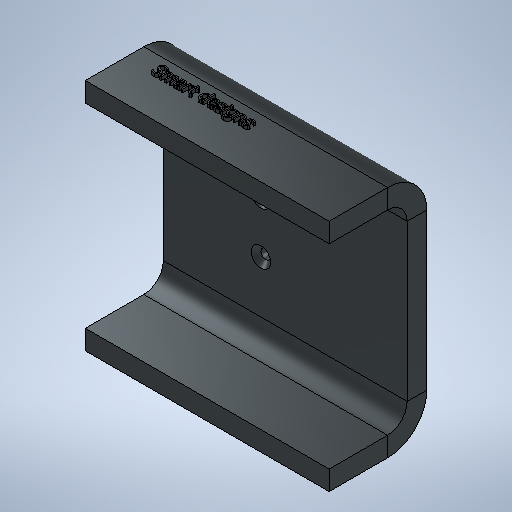
# Autodesk Inventor part: base
Saved by Autodesk Inventor 2025 (Build 290162010, 162A)
## iProperties
Created: 2024-06-06
Part Number: base
Material: Iron, Gray
Document SubType Name: Sheet Metal
Designer: ffogue
Density: 7.15 g/cm^3
Sheet Metal Rule: Default_mm
Appearance: Iron Gray
Author: ffogue
Autodesk Inventor part; units mm, degrees
note: some values were not read from the file. Chosen so that the rebuilt part matches the saved one: direction of "Bohrung2"; direction of "Emboss1".
ref_plane "YZ Plane" through (0, 0, 0) normal (1, 0, 0) x (0, 1, 0)
ref_plane "XZ Plane" through (0, 0, 0) normal (0, 1, 0) x (-1, 0, 0)
ref_plane "XY Plane" through (0, 0, 0) normal (0, 0, 1) x (1, 0, 0)
sketch "Skizze1" plane through (0, 0, 0) normal (0, 1, 0) x (-1, 0, 0)
  line L0 (37.5, -30) -> (-37.5, -30)
  line L1 (-37.5, -30) -> (-37.5, 30)
  line L2 (-37.5, 30) -> (37.5, 30)
  line L3 (37.5, 30) -> (37.5, -30)
  line L4 (37.5, -30) -> (-37.5, 30) construction
  line L5 (-37.5, -30) -> (37.5, 30) construction
  point P0 (0, 0)
  dimension "d0" = 75
  dimension "d1" = 60
  measures "d0" distance between parallel lines of L3 L1
  measures "d1" distance between parallel lines of L0 L2
extrude "Grobblech2" add sketch "Skizze1" along normal blind 6
sketch "Skizze2" plane through (-37.5, 0, -30) normal (0, 0, -1) x (-1, 0, 0)
  line L0 (-75, 0) -> (0, 0)
  line L1 (0, 0) -> (0, 24)
  line L2 (0, 24) -> (-75, 24)
  line L3 (-75, 24) -> (-75, 0)
  constraints: 6 end point, 1 horizontal, 1 perpendicular, 1 vertical
edge flange "Lasche1" height 30 angle 90 thickness 6 bend radius 6 thickness toward (0, 0, -1) relief tear relief width 6 relief depth 3 corner gap 6 corner form 0 edges at (0, 6, -30) (0, 6, 30) wall of the first edge with corners at (37.5, 0, -30) (-37.5, 0, -30) (-37.5, -24, -30) (37.5, -24, -30)
bend "Biegung1"
corner "Ecke1"
sketch "Skizze3" plane through (0, 0, 0) normal (0, 1, 0) x (1, 0, 0)
  line L0 (-37.5, -24) -> (-37.5, 24) projected
  line L1 (-37.5, 36) -> (37.5, 36) projected
  line L2 (-37.5, 24) -> (-37.5, 36) projected
  line L3 (37.5, 24) -> (-37.5, 24) projected
  line L4 (37.5, 24) -> (37.5, 36) projected
  point P0 (0, 0)
  point P1 (-7.5, 8)
  point P2 (-7.5, -8)
  dimension "d23" = 16
  dimension "d24" = 30
  dimension "d25" = 28
  constraints: 1 vertical alignment
  measures "d23" distance of point (-7.5, -8) point (-7.5, 8)
  measures "d24" distance from line of L0 point (-7.5, 8)
  measures "d25" distance from line of point (-7.5, 8) L1
hole "Bohrung2" at (-7.5, 0, -8) at (-7.5, 0, 8) direction (0, 1, 0) diameter 3 end up to surface countersink diameter 6 countersink angle 90
sketch "Sketch4" plane through (-37.5, -24, 36) normal (0, 0, 1) x (1, 0, 0)
  line L0 (8.2536, 15.3295) -> (38.2844, 15.3295) construction
  line L1 (38.2844, 15.3295) -> (38.2844, 10.6808) construction
  line L2 (38.2844, 10.6808) -> (8.2536, 10.6808) construction
  line L3 (8.2536, 10.6808) -> (8.2536, 15.3295) construction
  spline S0 degree 2 poles (9.5839, 11.6111) (9.2038, 11.6111) (8.6706, 11.77) (8.4352, 11.8834) knots 0 0 0 1 2 2 2
  line L4 (8.4352, 11.8834) -> (8.4352, 12.4677)
  line L5 (8.4352, 12.4677) -> (8.4692, 12.4677)
  spline S1 degree 2 poles (8.4692, 12.4677) (8.6989, 12.2521) (9.2804, 12.0139) (9.5498, 12.0139) knots 0 0 0 1 2 2 2
  spline S2 degree 2 poles (9.5498, 12.0139) (9.9356, 12.0139) (10.3298, 12.3344) (10.3298, 12.5982) knots 0 0 0 1 2 2 2
  spline S3 degree 2 poles (10.3298, 12.5982) (10.3298, 12.8081) (10.1228, 13.069) (9.8987, 13.1342) knots 0 0 0 1 2 2 2
  spline S4 degree 2 poles (9.8987, 13.1342) (9.737, 13.1796) (9.4676, 13.242) (9.2662, 13.2931) knots 0 0 0 1 2 2 2
  spline S5 degree 2 poles (9.2662, 13.2931) (9.0847, 13.3413) (8.7982, 13.4859) (8.6876, 13.6022) knots 0 0 0 1 2 2 2
  spline S6 degree 2 poles (8.6876, 13.6022) (8.5798, 13.7185) (8.4607, 14.0305) (8.4607, 14.2347) knots 0 0 0 1 2 2 2
  spline S7 degree 2 poles (8.4607, 14.2347) (8.4607, 14.6602) (9.1244, 15.2359) (9.6378, 15.2359) knots 0 0 0 1 2 2 2
  spline S8 degree 2 poles (9.6378, 15.2359) (9.9327, 15.2359) (10.4546, 15.1196) (10.6787, 15.009) knots 0 0 0 1 2 2 2
  line L6 (10.6787, 15.009) -> (10.6787, 14.4531)
  line L7 (10.6787, 14.4531) -> (10.6446, 14.4531)
  spline S9 degree 2 poles (10.6446, 14.4531) (10.4773, 14.6063) (9.9554, 14.8332) (9.669, 14.8332) knots 0 0 0 1 2 2 2
  spline S10 degree 2 poles (9.669, 14.8332) (9.3456, 14.8332) (8.9457, 14.5297) (8.9457, 14.2829) knots 0 0 0 1 2 2 2
  spline S11 degree 2 poles (8.9457, 14.2829) (8.9457, 14.0617) (9.1811, 13.7979) (9.4023, 13.7384) knots 0 0 0 1 2 2 2
  spline S12 degree 2 poles (9.4023, 13.7384) (9.5498, 13.6987) (9.9781, 13.5966) (10.1199, 13.554) knots 0 0 0 1 2 2 2
  spline S13 degree 2 poles (10.1199, 13.554) (10.4801, 13.4434) (10.8148, 12.9981) (10.8148, 12.6719) knots 0 0 0 1 2 2 2
  spline S14 degree 2 poles (10.8148, 12.6719) (10.8148, 12.4649) (10.6475, 12.0678) (10.4972, 11.9288) knots 0 0 0 1 2 2 2
  spline S15 degree 2 poles (10.4972, 11.9288) (10.3298, 11.7756) (9.9044, 11.6111) (9.5839, 11.6111) knots 0 0 0 1 2 2 2
  line L8 (14.2326, 11.6735) -> (14.2326, 13.1938)
  spline S16 degree 2 poles (14.2326, 13.1938) (14.2326, 13.3753) (14.2042, 13.6845) (14.1588, 13.7696) knots 0 0 0 1 2 2 2
  spline S17 degree 2 poles (14.1588, 13.7696) (14.1134, 13.8632) (13.9404, 13.9539) (13.7901, 13.9539) knots 0 0 0 1 2 2 2
  spline S18 degree 2 poles (13.7901, 13.9539) (13.654, 13.9539) (13.342, 13.7866) (13.1775, 13.6278) knots 0 0 0 1 2 2 2
  spline S19 degree 2 poles (13.1775, 13.6278) (13.1803, 13.588) (13.186, 13.4774) (13.186, 13.4037) knots 0 0 0 1 2 2 2
  line L9 (13.186, 13.4037) -> (13.186, 11.6735)
  line L10 (13.186, 11.6735) -> (12.7435, 11.6735)
  line L11 (12.7435, 11.6735) -> (12.7435, 13.1938)
  spline S20 degree 2 poles (12.7435, 13.1938) (12.7435, 13.3753) (12.7151, 13.6845) (12.6698, 13.7696) knots 0 0 0 1 2 2 2
  spline S21 degree 2 poles (12.6698, 13.7696) (12.6244, 13.8632) (12.4514, 13.9539) (12.301, 13.9539) knots 0 0 0 1 2 2 2
  spline S22 degree 2 poles (12.301, 13.9539) (12.1592, 13.9539) (11.8444, 13.7752) (11.6969, 13.6363) knots 0 0 0 1 2 2 2
  line L12 (11.6969, 13.6363) -> (11.6969, 11.6735)
  line L13 (11.6969, 11.6735) -> (11.2544, 11.6735)
  line L14 (11.2544, 11.6735) -> (11.2544, 14.3)
  line L15 (11.2544, 14.3) -> (11.6969, 14.3)
  line L16 (11.6969, 14.3) -> (11.6969, 14.0107)
  spline S23 degree 2 poles (11.6969, 14.0107) (11.8699, 14.1837) (12.2103, 14.3737) (12.4145, 14.3737) knots 0 0 0 1 2 2 2
  spline S24 degree 2 poles (12.4145, 14.3737) (12.6471, 14.3737) (13.0073, 14.161) (13.1009, 13.9199) knots 0 0 0 1 2 2 2
  spline S25 degree 2 poles (13.1009, 13.9199) (13.3023, 14.144) (13.6823, 14.3737) (13.9036, 14.3737) knots 0 0 0 1 2 2 2
  spline S26 degree 2 poles (13.9036, 14.3737) (14.0737, 14.3737) (14.3517, 14.2688) (14.4538, 14.1496) knots 0 0 0 1 2 2 2
  spline S27 degree 2 poles (14.4538, 14.1496) (14.5587, 14.0305) (14.675, 13.6731) (14.675, 13.4037) knots 0 0 0 1 2 2 2
  line L17 (14.675, 13.4037) -> (14.675, 11.6735)
  line L18 (14.675, 11.6735) -> (14.2326, 11.6735)
  spline S28 degree 2 poles (16.7597, 11.9515) (16.7058, 11.9118) (16.5243, 11.77) (16.4392, 11.7274) knots 0 0 0 1 2 2 2
  spline S29 degree 2 poles (16.4392, 11.7274) (16.3229, 11.665) (16.1045, 11.5998) (15.906, 11.5998) knots 0 0 0 1 2 2 2
  spline S30 degree 2 poles (15.906, 11.5998) (15.7443, 11.5998) (15.4522, 11.7218) (15.3416, 11.8324) knots 0 0 0 1 2 2 2
  spline S31 degree 2 poles (15.3416, 11.8324) (15.2366, 11.9402) (15.109, 12.2578) (15.109, 12.4337) knots 0 0 0 1 2 2 2
  spline S32 degree 2 poles (15.109, 12.4337) (15.109, 12.706) (15.3387, 13.0917) (15.5883, 13.2023) knots 0 0 0 1 2 2 2
  spline S33 degree 2 poles (15.5883, 13.2023) (15.8096, 13.3044) (16.4108, 13.381) (16.7597, 13.4008) knots 0 0 0 1 2 2 2
  line L19 (16.7597, 13.4008) -> (16.7597, 13.4859)
  spline S34 degree 2 poles (16.7597, 13.4859) (16.7597, 13.6391) (16.6661, 13.8291) (16.581, 13.883) knots 0 0 0 1 2 2 2
  spline S35 degree 2 poles (16.581, 13.883) (16.4959, 13.9369) (16.252, 13.9709) (16.1215, 13.9709) knots 0 0 0 1 2 2 2
  spline S36 degree 2 poles (16.1215, 13.9709) (15.9684, 13.9709) (15.5543, 13.8802) (15.3472, 13.7923) knots 0 0 0 1 2 2 2
  line L20 (15.3472, 13.7923) -> (15.3217, 13.7923)
  line L21 (15.3217, 13.7923) -> (15.3217, 14.2432)
  spline S37 degree 2 poles (15.3217, 14.2432) (15.4437, 14.2773) (15.9003, 14.3624) (16.1244, 14.3624) knots 0 0 0 1 2 2 2
  spline S38 degree 2 poles (16.1244, 14.3624) (16.3967, 14.3624) (16.7682, 14.2773) (16.9157, 14.1667) knots 0 0 0 1 2 2 2
  spline S39 degree 2 poles (16.9157, 14.1667) (17.0604, 14.0589) (17.2022, 13.7157) (17.2022, 13.4689) knots 0 0 0 1 2 2 2
  line L22 (17.2022, 13.4689) -> (17.2022, 11.6735)
  line L23 (17.2022, 11.6735) -> (16.7597, 11.6735)
  line L24 (16.7597, 11.6735) -> (16.7597, 11.9515)
  line L25 (16.7597, 12.3202) -> (16.7597, 13.0491)
  spline S40 degree 2 poles (16.7597, 13.0491) (16.6009, 13.035) (16.1215, 12.9867) (15.9712, 12.9414) knots 0 0 0 1 2 2 2
  spline S41 degree 2 poles (15.9712, 12.9414) (15.7954, 12.8875) (15.5656, 12.6634) (15.5656, 12.4649) knots 0 0 0 1 2 2 2
  spline S42 degree 2 poles (15.5656, 12.4649) (15.5656, 12.238) (15.8209, 12.0082) (16.0648, 12.0082) knots 0 0 0 1 2 2 2
  spline S43 degree 2 poles (16.0648, 12.0082) (16.2719, 12.0082) (16.6122, 12.1869) (16.7597, 12.3202) knots 0 0 0 1 2 2 2
  line L26 (19.216, 13.8263) -> (19.1933, 13.8263)
  spline S44 degree 2 poles (19.1933, 13.8263) (19.1422, 13.8405) (19.0316, 13.8461) (18.955, 13.8461) knots 0 0 0 1 2 2 2
  spline S45 degree 2 poles (18.955, 13.8461) (18.7763, 13.8461) (18.4246, 13.6902) (18.2658, 13.537) knots 0 0 0 1 2 2 2
  line L27 (18.2658, 13.537) -> (18.2658, 11.6735)
  line L28 (18.2658, 11.6735) -> (17.8233, 11.6735)
  line L29 (17.8233, 11.6735) -> (17.8233, 14.3)
  line L30 (17.8233, 14.3) -> (18.2658, 14.3)
  line L31 (18.2658, 14.3) -> (18.2658, 13.9085)
  spline S46 degree 2 poles (18.2658, 13.9085) (18.5069, 14.1241) (18.8671, 14.3) (19.0373, 14.3) knots 0 0 0 1 2 2 2
  spline S47 degree 2 poles (19.0373, 14.3) (19.1053, 14.3) (19.1734, 14.2943) (19.216, 14.2858) knots 0 0 0 1 2 2 2
  line L32 (19.216, 14.2858) -> (19.216, 13.8263)
  spline S48 degree 2 poles (20.3533, 11.6225) (19.9931, 11.6225) (19.5875, 12.0338) (19.5875, 12.4791) knots 0 0 0 1 2 2 2
  line L33 (19.5875, 12.4791) -> (19.5875, 13.9341)
  line L34 (19.5875, 13.9341) -> (19.2897, 13.9341)
  line L35 (19.2897, 13.9341) -> (19.2897, 14.3)
  line L36 (19.2897, 14.3) -> (19.5875, 14.3)
  line L37 (19.5875, 14.3) -> (19.5875, 15.0544)
  line L38 (19.5875, 15.0544) -> (20.03, 15.0544)
  line L39 (20.03, 15.0544) -> (20.03, 14.3)
  line L40 (20.03, 14.3) -> (20.844, 14.3)
  line L41 (20.844, 14.3) -> (20.844, 13.9341)
  line L42 (20.844, 13.9341) -> (20.03, 13.9341)
  line L43 (20.03, 13.9341) -> (20.03, 12.6833)
  spline S49 degree 2 poles (20.03, 12.6833) (20.03, 12.4847) (20.0442, 12.2663) (20.0924, 12.1727) knots 0 0 0 1 2 2 2
  spline S50 degree 2 poles (20.0924, 12.1727) (20.1321, 12.0905) (20.3108, 12.0082) (20.4639, 12.0082) knots 0 0 0 1 2 2 2
  spline S51 degree 2 poles (20.4639, 12.0082) (20.5717, 12.0082) (20.7731, 12.0735) (20.8185, 12.0933) knots 0 0 0 1 2 2 2
  line L44 (20.8185, 12.0933) -> (20.844, 12.0933)
  line L45 (20.844, 12.0933) -> (20.844, 11.6962)
  spline S52 degree 2 poles (20.844, 11.6962) (20.7192, 11.6622) (20.4639, 11.6225) (20.3533, 11.6225) knots 0 0 0 1 2 2 2
  line L46 (24.6929, 11.6735) -> (24.2504, 11.6735)
  line L47 (24.2504, 11.6735) -> (24.2504, 11.9402)
  spline S53 degree 2 poles (24.2504, 11.9402) (24.1483, 11.8551) (23.998, 11.7416) (23.8959, 11.6934) knots 0 0 0 1 2 2 2
  spline S54 degree 2 poles (23.8959, 11.6934) (23.8023, 11.648) (23.6009, 11.5998) (23.4676, 11.5998) knots 0 0 0 1 2 2 2
  spline S55 degree 2 poles (23.4676, 11.5998) (23.252, 11.5998) (22.889, 11.7785) (22.7613, 11.9515) knots 0 0 0 1 2 2 2
  spline S56 degree 2 poles (22.7613, 11.9515) (22.6337, 12.1245) (22.4919, 12.635) (22.4919, 12.9669) knots 0 0 0 1 2 2 2
  spline S57 degree 2 poles (22.4919, 12.9669) (22.4919, 13.3129) (22.6706, 13.8178) (22.8266, 14.0078) knots 0 0 0 1 2 2 2
  spline S58 degree 2 poles (22.8266, 14.0078) (22.9712, 14.178) (23.3768, 14.3737) (23.6009, 14.3737) knots 0 0 0 1 2 2 2
  spline S59 degree 2 poles (23.6009, 14.3737) (23.7966, 14.3737) (24.0887, 14.2858) (24.2504, 14.195) knots 0 0 0 1 2 2 2
  line L48 (24.2504, 14.195) -> (24.2504, 15.3295)
  line L49 (24.2504, 15.3295) -> (24.6929, 15.3295)
  line L50 (24.6929, 15.3295) -> (24.6929, 11.6735)
  line L51 (24.2504, 12.3117) -> (24.2504, 13.8291)
  spline S60 degree 2 poles (24.2504, 13.8291) (24.0859, 13.9085) (23.8249, 13.9681) (23.6746, 13.9681) knots 0 0 0 1 2 2 2
  spline S61 degree 2 poles (23.6746, 13.9681) (23.3343, 13.9681) (22.9485, 13.4576) (22.9485, 12.9754) knots 0 0 0 1 2 2 2
  spline S62 degree 2 poles (22.9485, 12.9754) (22.9485, 12.5102) (23.2435, 12.0196) (23.5697, 12.0196) knots 0 0 0 1 2 2 2
  spline S63 degree 2 poles (23.5697, 12.0196) (23.7427, 12.0196) (24.0944, 12.1784) (24.2504, 12.3117) knots 0 0 0 1 2 2 2
  spline S64 degree 2 poles (26.4741, 11.614) (25.8444, 11.614) (25.1523, 12.3202) (25.1523, 12.9726) knots 0 0 0 1 2 2 2
  spline S65 degree 2 poles (25.1523, 12.9726) (25.1523, 13.6136) (25.8245, 14.3737) (26.3663, 14.3737) knots 0 0 0 1 2 2 2
  spline S66 degree 2 poles (26.3663, 14.3737) (26.6102, 14.3737) (26.9874, 14.2319) (27.1264, 14.0816) knots 0 0 0 1 2 2 2
  spline S67 degree 2 poles (27.1264, 14.0816) (27.2682, 13.9312) (27.4185, 13.4973) (27.4185, 13.1825) knots 0 0 0 1 2 2 2
  line L52 (27.4185, 13.1825) -> (27.4185, 12.9414)
  line L53 (27.4185, 12.9414) -> (25.6005, 12.9414)
  spline S68 degree 2 poles (25.6005, 12.9414) (25.6005, 12.4847) (26.06, 11.9997) (26.4684, 11.9997) knots 0 0 0 1 2 2 2
  spline S69 degree 2 poles (26.4684, 11.9997) (26.613, 11.9997) (26.8938, 12.0649) (27.0073, 12.116) knots 0 0 0 1 2 2 2
  spline S70 degree 2 poles (27.0073, 12.116) (27.1264, 12.1727) (27.2909, 12.272) (27.3448, 12.3174) knots 0 0 0 1 2 2 2
  line L54 (27.3448, 12.3174) -> (27.3703, 12.3174)
  line L55 (27.3703, 12.3174) -> (27.3703, 11.8352)
  spline S71 degree 2 poles (27.3703, 11.8352) (27.2937, 11.804) (27.0612, 11.7132) (26.9704, 11.6877) knots 0 0 0 1 2 2 2
  spline S72 degree 2 poles (26.9704, 11.6877) (26.8428, 11.6508) (26.6329, 11.614) (26.4741, 11.614) knots 0 0 0 1 2 2 2
  spline S73 degree 2 poles (26.9874, 13.2789) (26.9818, 13.4576) (26.908, 13.7185) (26.8371, 13.8064) knots 0 0 0 1 2 2 2
  spline S74 degree 2 poles (26.8371, 13.8064) (26.7605, 13.9057) (26.5194, 14.0107) (26.3408, 14.0107) knots 0 0 0 1 2 2 2
  spline S75 degree 2 poles (26.3408, 14.0107) (26.1649, 14.0107) (25.9181, 13.9057) (25.816, 13.8036) knots 0 0 0 1 2 2 2
  spline S76 degree 2 poles (25.816, 13.8036) (25.7168, 13.6987) (25.6147, 13.4462) (25.6005, 13.2789) knots 0 0 0 1 2 2 2
  line L56 (25.6005, 13.2789) -> (26.9874, 13.2789)
  spline S77 degree 2 poles (28.5758, 11.6111) (28.312, 11.6111) (27.8553, 11.753) (27.705, 11.8324) knots 0 0 0 1 2 2 2
  line L57 (27.705, 11.8324) -> (27.705, 12.3287)
  line L58 (27.705, 12.3287) -> (27.7277, 12.3287)
  spline S78 degree 2 poles (27.7277, 12.3287) (27.7844, 12.2833) (27.9376, 12.1756) (28.0652, 12.116) knots 0 0 0 1 2 2 2
  spline S79 degree 2 poles (28.0652, 12.116) (28.1758, 12.0621) (28.4481, 11.9827) (28.5928, 11.9827) knots 0 0 0 1 2 2 2
  spline S80 degree 2 poles (28.5928, 11.9827) (28.6977, 11.9827) (28.9388, 12.0309) (28.9955, 12.0706) knots 0 0 0 1 2 2 2
  spline S81 degree 2 poles (28.9955, 12.0706) (29.0778, 12.1245) (29.1515, 12.2465) (29.1515, 12.3713) knots 0 0 0 1 2 2 2
  spline S82 degree 2 poles (29.1515, 12.3713) (29.1515, 12.5273) (28.9813, 12.6889) (28.763, 12.7428) knots 0 0 0 1 2 2 2
  spline S83 degree 2 poles (28.763, 12.7428) (28.6779, 12.7627) (28.4056, 12.8194) (28.2893, 12.8506) knots 0 0 0 1 2 2 2
  spline S84 degree 2 poles (28.2893, 12.8506) (27.9886, 12.9385) (27.7164, 13.3016) (27.7164, 13.5597) knots 0 0 0 1 2 2 2
  spline S85 degree 2 poles (27.7164, 13.5597) (27.7164, 13.9171) (28.2524, 14.3624) (28.6949, 14.3624) knots 0 0 0 1 2 2 2
  spline S86 degree 2 poles (28.6949, 14.3624) (28.9133, 14.3624) (29.3557, 14.2546) (29.5061, 14.1723) knots 0 0 0 1 2 2 2
  line L59 (29.5061, 14.1723) -> (29.5061, 13.6987)
  line L60 (29.5061, 13.6987) -> (29.4834, 13.6987)
  spline S87 degree 2 poles (29.4834, 13.6987) (29.3132, 13.8348) (28.8991, 13.9908) (28.6864, 13.9908) knots 0 0 0 1 2 2 2
  spline S88 degree 2 poles (28.6864, 13.9908) (28.468, 13.9908) (28.1673, 13.8064) (28.1673, 13.6221) knots 0 0 0 1 2 2 2
  spline S89 degree 2 poles (28.1673, 13.6221) (28.1673, 13.4547) (28.346, 13.2931) (28.5446, 13.242) knots 0 0 0 1 2 2 2
  spline S90 degree 2 poles (28.5446, 13.242) (28.641, 13.2165) (28.8849, 13.1654) (29.0182, 13.1342) knots 0 0 0 1 2 2 2
  spline S91 degree 2 poles (29.0182, 13.1342) (29.3075, 13.0605) (29.6025, 12.723) (29.6025, 12.4308) knots 0 0 0 1 2 2 2
  spline S92 degree 2 poles (29.6025, 12.4308) (29.6025, 12.2607) (29.4692, 11.96) (29.3387, 11.8494) knots 0 0 0 1 2 2 2
  spline S93 degree 2 poles (29.3387, 11.8494) (29.1997, 11.7331) (28.8452, 11.6111) (28.5758, 11.6111) knots 0 0 0 1 2 2 2
  line L61 (30.4647, 11.6735) -> (30.0223, 11.6735)
  line L62 (30.0223, 11.6735) -> (30.0223, 14.3)
  line L63 (30.0223, 14.3) -> (30.4647, 14.3)
  line L64 (30.4647, 14.3) -> (30.4647, 11.6735)
  line L65 (30.4959, 14.7367) -> (29.9939, 14.7367)
  line L66 (29.9939, 14.7367) -> (29.9939, 15.1962)
  line L67 (29.9939, 15.1962) -> (30.4959, 15.1962)
  line L68 (30.4959, 15.1962) -> (30.4959, 14.7367)
  spline S94 degree 2 poles (31.2078, 11.2538) (31.2532, 11.2339) (31.4262, 11.1715) (31.5369, 11.146) knots 0 0 0 1 2 2 2
  spline S95 degree 2 poles (31.5369, 11.146) (31.6588, 11.1148) (31.8659, 11.0779) (31.9878, 11.0779) knots 0 0 0 1 2 2 2
  spline S96 degree 2 poles (31.9878, 11.0779) (32.192, 11.0779) (32.4757, 11.1857) (32.5551, 11.2821) knots 0 0 0 1 2 2 2
  spline S97 degree 2 poles (32.5551, 11.2821) (32.6317, 11.3786) (32.6912, 11.631) (32.6912, 11.7927) knots 0 0 0 1 2 2 2
  line L69 (32.6912, 11.7927) -> (32.6912, 12.0224)
  spline S98 degree 2 poles (32.6912, 12.0224) (32.5125, 11.8664) (32.1694, 11.7189) (31.9113, 11.7189) knots 0 0 0 1 2 2 2
  spline S99 degree 2 poles (31.9113, 11.7189) (31.4631, 11.7189) (30.9327, 12.3855) (30.9327, 13.0123) knots 0 0 0 1 2 2 2
  spline S100 degree 2 poles (30.9327, 13.0123) (30.9327, 13.3385) (31.1171, 13.8433) (31.2702, 14.022) knots 0 0 0 1 2 2 2
  spline S101 degree 2 poles (31.2702, 14.022) (31.4177, 14.1893) (31.8233, 14.3737) (32.0389, 14.3737) knots 0 0 0 1 2 2 2
  spline S102 degree 2 poles (32.0389, 14.3737) (32.2431, 14.3737) (32.5409, 14.2773) (32.6912, 14.1893) knots 0 0 0 1 2 2 2
  line L70 (32.6912, 14.1893) -> (32.7168, 14.3)
  line L71 (32.7168, 14.3) -> (33.1337, 14.3)
  line L72 (33.1337, 14.3) -> (33.1337, 11.9742)
  spline S103 degree 2 poles (33.1337, 11.9742) (33.1337, 11.3048) (32.5523, 10.6808) (31.9538, 10.6808) knots 0 0 0 1 2 2 2
  spline S104 degree 2 poles (31.9538, 10.6808) (31.7609, 10.6808) (31.3582, 10.7432) (31.1852, 10.7943) knots 0 0 0 1 2 2 2
  line L73 (31.1852, 10.7943) -> (31.1852, 11.2538)
  line L74 (31.1852, 11.2538) -> (31.2078, 11.2538)
  line L75 (32.6912, 12.3855) -> (32.6912, 13.8291)
  spline S105 degree 2 poles (32.6912, 13.8291) (32.5267, 13.9085) (32.2488, 13.9766) (32.1098, 13.9766) knots 0 0 0 1 2 2 2
  spline S106 degree 2 poles (32.1098, 13.9766) (31.7751, 13.9766) (31.3894, 13.4831) (31.3894, 13.0208) knots 0 0 0 1 2 2 2
  spline S107 degree 2 poles (31.3894, 13.0208) (31.3894, 12.584) (31.6815, 12.1273) (32.0105, 12.1273) knots 0 0 0 1 2 2 2
  spline S108 degree 2 poles (32.0105, 12.1273) (32.1835, 12.1273) (32.5466, 12.2635) (32.6912, 12.3855) knots 0 0 0 1 2 2 2
  line L76 (35.8367, 11.6735) -> (35.3942, 11.6735)
  line L77 (35.3942, 11.6735) -> (35.3942, 13.1711)
  spline S109 degree 2 poles (35.3942, 13.1711) (35.3942, 13.3526) (35.3602, 13.6646) (35.3091, 13.7582) knots 0 0 0 1 2 2 2
  spline S110 degree 2 poles (35.3091, 13.7582) (35.2553, 13.8575) (35.0624, 13.9539) (34.8979, 13.9539) knots 0 0 0 1 2 2 2
  spline S111 degree 2 poles (34.8979, 13.9539) (34.7334, 13.9539) (34.3845, 13.7781) (34.2172, 13.6363) knots 0 0 0 1 2 2 2
  line L78 (34.2172, 13.6363) -> (34.2172, 11.6735)
  line L79 (34.2172, 11.6735) -> (33.7747, 11.6735)
  line L80 (33.7747, 11.6735) -> (33.7747, 14.3)
  line L81 (33.7747, 14.3) -> (34.2172, 14.3)
  line L82 (34.2172, 14.3) -> (34.2172, 14.0078)
  spline S112 degree 2 poles (34.2172, 14.0078) (34.4157, 14.1865) (34.7986, 14.3737) (35.0142, 14.3737) knots 0 0 0 1 2 2 2
  spline S113 degree 2 poles (35.0142, 14.3737) (35.3999, 14.3737) (35.8367, 13.8632) (35.8367, 13.3782) knots 0 0 0 1 2 2 2
  line L83 (35.8367, 13.3782) -> (35.8367, 11.6735)
  spline S114 degree 2 poles (37.1669, 11.6111) (36.9031, 11.6111) (36.4465, 11.753) (36.2962, 11.8324) knots 0 0 0 1 2 2 2
  line L84 (36.2962, 11.8324) -> (36.2962, 12.3287)
  line L85 (36.2962, 12.3287) -> (36.3189, 12.3287)
  spline S115 degree 2 poles (36.3189, 12.3287) (36.3756, 12.2833) (36.5288, 12.1756) (36.6564, 12.116) knots 0 0 0 1 2 2 2
  spline S116 degree 2 poles (36.6564, 12.116) (36.767, 12.0621) (37.0393, 11.9827) (37.1839, 11.9827) knots 0 0 0 1 2 2 2
  spline S117 degree 2 poles (37.1839, 11.9827) (37.2889, 11.9827) (37.53, 12.0309) (37.5867, 12.0706) knots 0 0 0 1 2 2 2
  spline S118 degree 2 poles (37.5867, 12.0706) (37.669, 12.1245) (37.7427, 12.2465) (37.7427, 12.3713) knots 0 0 0 1 2 2 2
  spline S119 degree 2 poles (37.7427, 12.3713) (37.7427, 12.5273) (37.5725, 12.6889) (37.3541, 12.7428) knots 0 0 0 1 2 2 2
  spline S120 degree 2 poles (37.3541, 12.7428) (37.269, 12.7627) (36.9967, 12.8194) (36.8805, 12.8506) knots 0 0 0 1 2 2 2
  spline S121 degree 2 poles (36.8805, 12.8506) (36.5798, 12.9385) (36.3075, 13.3016) (36.3075, 13.5597) knots 0 0 0 1 2 2 2
  spline S122 degree 2 poles (36.3075, 13.5597) (36.3075, 13.9171) (36.8436, 14.3624) (37.286, 14.3624) knots 0 0 0 1 2 2 2
  spline S123 degree 2 poles (37.286, 14.3624) (37.5044, 14.3624) (37.9469, 14.2546) (38.0972, 14.1723) knots 0 0 0 1 2 2 2
  line L86 (38.0972, 14.1723) -> (38.0972, 13.6987)
  line L87 (38.0972, 13.6987) -> (38.0745, 13.6987)
  spline S124 degree 2 poles (38.0745, 13.6987) (37.9044, 13.8348) (37.4903, 13.9908) (37.2775, 13.9908) knots 0 0 0 1 2 2 2
  spline S125 degree 2 poles (37.2775, 13.9908) (37.0591, 13.9908) (36.7585, 13.8064) (36.7585, 13.6221) knots 0 0 0 1 2 2 2
  spline S126 degree 2 poles (36.7585, 13.6221) (36.7585, 13.4547) (36.9372, 13.2931) (37.1357, 13.242) knots 0 0 0 1 2 2 2
  spline S127 degree 2 poles (37.1357, 13.242) (37.2322, 13.2165) (37.4761, 13.1654) (37.6094, 13.1342) knots 0 0 0 1 2 2 2
  spline S128 degree 2 poles (37.6094, 13.1342) (37.8987, 13.0605) (38.1937, 12.723) (38.1937, 12.4308) knots 0 0 0 1 2 2 2
  spline S129 degree 2 poles (38.1937, 12.4308) (38.1937, 12.2607) (38.0604, 11.96) (37.9299, 11.8494) knots 0 0 0 1 2 2 2
  spline S130 degree 2 poles (37.9299, 11.8494) (37.7909, 11.7331) (37.4364, 11.6111) (37.1669, 11.6111) knots 0 0 0 1 2 2 2
  point P0 (37.5, 24)
  constraints: 2 other
emboss "Emboss1" sketch "Sketch4" operation add depth 1 direction (0, 0, -1)
equation "\"Abstandsgröße\" = Stärke"
equation "\"d5\" = Stärke"
equation "\"d6\" = BreiteBiegungsfreistellung"
equation "\"d7\" = TiefeBiegungsfreistellung"
equation "\"d8\" = MinimalRest"
equation "\"d9\" = Übergangsradius"
equation "\"d12\" = Biegeradius"
equation "\"d13\" = GrößeEckenfreistellung"
equation "\"d14\" = Abstandsgröße"
equation "\"d15\" = JacobiRadiusGröße"
equation "\"Biegeradius\" = Stärke"
equation "\"BreiteBiegungsfreistellung\" = Stärke"
equation "\"TiefeBiegungsfreistellung\" = 0.5 * Stärke"
equation "\"GrößeEckenfreistellung\" = 4 * Stärke"
equation "\"MinimalRest\" = 2 * Stärke"
equation "\"Übergangsradius\" = Biegeradius"
equation "\"JacobiRadiusGröße\" = Biegeradius"
equation "\"Stärke\" = 6"
